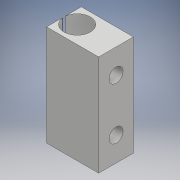
# Autodesk Inventor part: x_holder
Saved by Autodesk Inventor 2017 (Build 210142000, 142)
## iProperties
Part Number: x_holder
Material: Типовые
Document SubType Name: Modeling
Designer: Tolya
Density: 1 g/cm^3
Appearance: По умолчанию
Author: Tolya
Autodesk Inventor part; units mm, degrees
ref_plane "YZ Plane" through (0, 0, 0) normal (1, 0, 0) x (0, 1, 0)
ref_plane "XZ Plane" through (0, 0, 0) normal (0, 1, 0) x (-1, 0, 0)
ref_plane "XY Plane" through (0, 0, 0) normal (0, 0, 1) x (1, 0, 0)
sketch "Эскиз1" plane through (0, 0, 0) normal (0, 0, 1) x (1, 0, 0)
  line L0 (0, 0) -> (30, 0)
  line L1 (30, 0) -> (30, 20)
  line L2 (30, 20) -> (0, 20)
  arc A0 (0.0661, 9) -> (0.0661, 11) centre (7.6, 10) ccw
  line L3 (0.0661, 11) -> (0, 11)
  line L4 (0.0661, 9) -> (0, 9)
  line L5 (0, 20) -> (0, 11)
  line L6 (0, 9) -> (0, 0)
  dimension "d0" = 30
  dimension "d1" = 20
  constraints: 14 end point, 5 perpendicular, 3 parallel, 2 point on circle, 1 centre point, 1 horizontal
  measures "d0" distance of L2.end L1.end
  measures "d1" distance of L1.end L0.end
extrude "Выдавливание1" add sketch "Эскиз1" along normal blind 58
sketch "Эскиз2" plane through (30, 0, 0) normal (1, 0, 0) x (0, 0, -1)
  circle A0 centre (-14.05, 10) radius 4.05
  line L0 (0, 20) -> (-58, 20) projected
  line L1 (-29, 20) -> (-29, 0)
  circle A1 centre (-43.95, 10) radius 4.05
  point P0 (0, 0)
  dimension "d4" = 8.1
  constraints: 2 centre point, 2 end point, 1 midpoint, 1 symmetric about line, 1 vertical, 1 other
  measures "d4" diameter of A0
extrude "Выдавливание2" cut sketch "Эскиз2" against normal blind 10
